Autodesk Inventor part; units mm, degrees
(part 2 of 2)
  line L146 (-17.2139, 92.4267) -> (-17.7029, 92.4267)
  line L147 (-17.7029, 92.4267) -> (-17.7029, 93.0096)
  line L148 (-20.1977, 93.0096) -> (-18.318, 93.0096)
  line L149 (-18.318, 93.0096) -> (-18.318, 92.5774)
  spline S117 degree 2 poles (-18.318, 92.5774) (-18.5205, 92.3872) (-18.8811, 92.034) (-19.054, 91.8438) knots 0 0 0 1 2 2 2
  spline S118 degree 2 poles (-19.054, 91.8438) (-19.4023, 91.4609) (-19.6567, 91.0015) (-19.6567, 90.757) knots 0 0 0 1 2 2 2
  spline S119 degree 2 poles (-19.6567, 90.757) (-19.6567, 90.6285) (-19.5777, 90.4359) (-19.5061, 90.3741) knots 0 0 0 1 2 2 2
  spline S120 degree 2 poles (-19.5061, 90.3741) (-19.4344, 90.3124) (-19.2467, 90.2506) (-19.1331, 90.2506) knots 0 0 0 1 2 2 2
  spline S121 degree 2 poles (-19.1331, 90.2506) (-19.0244, 90.2506) (-18.8021, 90.305) (-18.7008, 90.347) knots 0 0 0 1 2 2 2
  spline S122 degree 2 poles (-18.7008, 90.347) (-18.6144, 90.3815) (-18.4538, 90.4803) (-18.4044, 90.5149) knots 0 0 0 1 2 2 2
  line L150 (-18.4044, 90.5149) -> (-18.3822, 90.5149)
  line L151 (-18.3822, 90.5149) -> (-18.3822, 90.0802)
  spline S123 degree 2 poles (-18.3822, 90.0802) (-18.5082, 90.0184) (-18.9602, 89.8974) (-19.1627, 89.8974) knots 0 0 0 1 2 2 2
  spline S124 degree 2 poles (-19.1627, 89.8974) (-19.59, 89.8974) (-20.0717, 90.3494) (-20.0717, 90.7347) knots 0 0 0 1 2 2 2
  spline S125 degree 2 poles (-20.0717, 90.7347) (-20.0717, 90.9151) (-19.9877, 91.2164) (-19.9136, 91.3448) knots 0 0 0 1 2 2 2
  spline S126 degree 2 poles (-19.9136, 91.3448) (-19.8395, 91.4782) (-19.6246, 91.74) (-19.5061, 91.866) knots 0 0 0 1 2 2 2
  spline S127 degree 2 poles (-19.5061, 91.866) (-19.3134, 92.076) (-18.8416, 92.5255) (-18.7008, 92.6564) knots 0 0 0 1 2 2 2
  line L152 (-18.7008, 92.6564) -> (-20.1977, 92.6564)
  line L153 (-20.1977, 92.6564) -> (-20.1977, 93.0096)
  spline S128 degree 2 poles (-22.4528, 92.0414) (-22.4528, 92.2612) (-22.312, 92.6367) (-22.1836, 92.775) knots 0 0 0 1 2 2 2
  spline S129 degree 2 poles (-22.1836, 92.775) (-22.0551, 92.9133) (-21.6723, 93.0738) (-21.4351, 93.0738) knots 0 0 0 1 2 2 2
  spline S130 degree 2 poles (-21.4351, 93.0738) (-21.2178, 93.0738) (-20.7929, 92.9775) (-20.6373, 92.9009) knots 0 0 0 1 2 2 2
  line L154 (-20.6373, 92.9009) -> (-20.6373, 92.4687)
  line L155 (-20.6373, 92.4687) -> (-20.667, 92.4687)
  spline S131 degree 2 poles (-20.667, 92.4687) (-20.7139, 92.5033) (-20.8893, 92.5922) (-20.9955, 92.6317) knots 0 0 0 1 2 2 2
  spline S132 degree 2 poles (-20.9955, 92.6317) (-21.1165, 92.6737) (-21.3166, 92.7206) (-21.4426, 92.7206) knots 0 0 0 1 2 2 2
  spline S133 degree 2 poles (-21.4426, 92.7206) (-21.5661, 92.7206) (-21.7982, 92.6317) (-21.8822, 92.5354) knots 0 0 0 1 2 2 2
  spline S134 degree 2 poles (-21.8822, 92.5354) (-21.9588, 92.444) (-22.0378, 92.2019) (-22.0378, 92.0389) knots 0 0 0 1 2 2 2
  spline S135 degree 2 poles (-22.0378, 92.0389) (-22.0378, 91.8759) (-21.9489, 91.6684) (-21.8649, 91.5992) knots 0 0 0 1 2 2 2
  spline S136 degree 2 poles (-21.8649, 91.5992) (-21.7785, 91.5227) (-21.5216, 91.4585) (-21.366, 91.4585) knots 0 0 0 1 2 2 2
  spline S137 degree 2 poles (-21.366, 91.4585) (-21.198, 91.4585) (-20.8646, 91.5103) (-20.7633, 91.5326) knots 0 0 0 1 2 2 2
  line L156 (-20.7633, 91.5326) -> (-20.7633, 89.9616)
  line L157 (-20.7633, 89.9616) -> (-22.4355, 89.9616)
  line L158 (-22.4355, 89.9616) -> (-22.4355, 90.3198)
  line L159 (-22.4355, 90.3198) -> (-21.156, 90.3198)
  line L160 (-21.156, 90.3198) -> (-21.156, 91.1324)
  spline S138 degree 2 poles (-21.156, 91.1324) (-21.2301, 91.1225) (-21.3734, 91.1151) (-21.4327, 91.1151) knots 0 0 0 1 2 2 2
  spline S139 degree 2 poles (-21.4327, 91.1151) (-21.6673, 91.1151) (-21.9909, 91.1917) (-22.1391, 91.3053) knots 0 0 0 1 2 2 2
  spline S140 degree 2 poles (-22.1391, 91.3053) (-22.2898, 91.4189) (-22.4528, 91.7647) (-22.4528, 92.0414) knots 0 0 0 1 2 2 2
  point P0 (-47.5, 53.2457)
  constraints: 2 other
extrude "Extrusion47" cut sketch "Sketch58" against normal blind 1.5
sketch "Sketch59" plane through (69.5, 80.5, 0) normal (0, 0, -1) x (-1, 0, 0)
  line L0 (124.232, -148.2248) -> (124.232, -65.5994) projected
  line L1 (124.232, -131.7625) -> (22.225, -131.7625)
  line L2 (22.225, -144.4625) -> (124.232, -144.4625)
  line L3 (124.232, -144.4625) -> (124.232, -131.7625)
  line L4 (22.225, -144.4625) -> (19.05, -144.4625)
  line L5 (19.05, -144.4625) -> (19.05, -131.7625)
  line L6 (19.05, -131.7625) -> (22.225, -131.7625)
  point P0 (69.5, -80.5)
  point P1 (22.225, -131.7625)
  constraints: 12 end point, 2 horizontal, 2 parallel, 1 perpendicular, 1 point on line
extrude "Extrusion48" add sketch "Sketch59" against normal blind 1
sketch "Sketch61" plane through (-54.732, -66.7303, 5) normal (-1, 0, 0) x (0, 0, 1)
  point P0 (-5, 66.7303)
sketch "Sketch63" plane through (-54.732, -66.7303, 5) normal (-1, 0, 0) x (0, 0, 1)
  line L0 (0, 0) -> (32.8849, -46.9646) projected
  line L1 (32.8849, -46.9646) -> (72.2795, -19.3802)
  line L2 (72.2795, -19.3802) -> (86.4989, -39.6875)
  line L3 (86.4989, -39.6875) -> (32.8849, -46.9646)
  point P0 (-5, 66.7303)
  constraints: 6 end point, 2 perpendicular
extrude "Extrusion50" cut sketch "Sketch63" against normal blind 155.1
sketch "Sketch64" plane through (-54.732, -87.3593, 75.4961) normal (0, -0.819152, 0.5735764) x (1, 0, 0)
  line L0 (6, 0) -> (6, -45.9148) projected
  line L1 (0, -45.9148) -> (0, 21.0852) projected
  line L2 (0, 0) -> (0, -5)
  line L3 (0, -5) -> (3.5, -5)
  line L4 (3.5, -5) -> (0.6132, 0)
  line L5 (0, 0) -> (0, 0.5341)
  line L6 (0, 0.5341) -> (0.3049, 0.5341)
  line L7 (0.3049, 0.5341) -> (0.6312, -0.0311)
  line L8 (98.464, 0) -> (104.464, 0) projected
  line L9 (104.464, 0) -> (104.464, -5)
  line L10 (104.464, 21.0852) -> (104.464, -45.9148) projected
  line L11 (104.464, -5) -> (100.964, -5)
  line L12 (100.964, -5) -> (103.8508, 0)
  line L13 (103.8508, 0) -> (104.1591, 0.5341)
  line L14 (104.1591, 0.5341) -> (104.464, 0.5341)
  line L15 (104.464, 0.5341) -> (104.464, -0.2668)
  point P0 (0.6132, 0)
  dimension "d248" = 5
  dimension "d249" = 3.5
  dimension "d250" = 60
  dimension "d251" = 5
  dimension "d252" = 3.5
  dimension "d253" = 60
  constraints: 24 end point, 7 point on line, 2 horizontal, 2 perpendicular
  measures "d248" distance of L2.start L2.end
  measures "d249" distance of L2.end L3.end
  measures "d250" angle of L4 L3
  measures "d251" distance of L8.end L9.end
  measures "d252" distance of L9.end L11.end
  measures "d253" angle of L12 L11
extrude "Extrusion51" cut sketch "Sketch64" against normal blind 100.764
sketch "Sketch65" plane through (47.5, -63.2207, 2.5425) normal (0, -0.5735764, -0.819152) x (-1, 0, 0)
  circle A0 centre (74.6125, -57.15) radius 2 projected
  circle A1 centre (74.6125, -57.15) radius 5
  circle A2 centre (84.6125, -33.45) radius 2 projected
  circle A3 centre (84.6125, -33.45) radius 5
  circle A4 centre (64.6125, -33.45) radius 2 projected
  circle A5 centre (64.6125, -33.45) radius 5
  point P0 (47.5, 53.2457)
  dimension "d254" = 10
  dimension "d255" = 10
  dimension "d256" = 10
  constraints: 3 centre point, 3 coincident
  measures "d254" diameter of A1
  measures "d255" diameter of A3
  measures "d256" diameter of A5
extrude "Extrusion52" cut sketch "Sketch65" against normal blind 3 contours A1 | A2 | A3 | A4 | A5
sketch "Sketch66" plane through (-48.732, -55.8368, 7.1384) normal (0, 0.819152, -0.5735764) x (1, 0, 0)
  line L0 (42.232, 0) -> (42.232, -16) projected
  line L1 (0, 0) -> (42.232, 0) projected
  line L2 (0, -16) -> (0, 0)
  line L3 (0, 0) -> (42.232, 0)
  line L4 (42.232, 0) -> (42.232, -16)
  arc A0 (34.925, -16) -> (9.0575, -16) centre (21.9913, -30.5193) ccw projected
  arc A1 (34.925, -16) -> (9.0575, -16) centre (21.9913, -30.5193) ccw
  line L5 (42.232, -16) -> (34.925, -16)
  line L6 (9.0575, -16) -> (0, -16)
  point P0 (48.732, -26.1792)
  constraints: 10 end point, 4 point on circle, 3 parallel, 2 horizontal, 2 perpendicular, 1 centre point
extrude "Extrusion53" add sketch "Sketch66" along normal blind 2
sketch "Sketch67" plane through (47.5, -58.6321, 9.0958) normal (0, 0.5735764, 0.819152) x (1, 0, 0)
  line L0 (-96.232, 5.4125) -> (-96.232, 15.858) projected
  line L1 (-3.768, -61.6176) -> (-3.768, 39.1469) projected
  line L2 (-3.768, 5.4125) -> (-3.768, 15.875)
  line L3 (-3.768, 15.875) -> (-96.232, 15.875)
  line L4 (-96.232, 15.875) -> (-96.232, 5.4125)
  line L5 (-3.768, 10.6437) -> (-96.232, 10.6437)
  point P0 (-47.5, 53.2457)
  point P1 (-96.232, 15.858)
  point P2 (-3.768, 10.6437)
  constraints: 8 end point, 2 midpoint, 1 parallel, 1 point on line
extrude "Extrusion54" add sketch "Sketch67" along normal blind 50
sketch "Sketch70" plane through (-48.732, -45.6281, -0.0098) normal (0, 0.819152, -0.5735764) x (1, 0, 0)
  line L0 (92.464, -37.9148) -> (92.464, -50) projected
  line L1 (0, -0.0119) -> (0, -60) projected
  line L2 (92.464, -50) -> (0, -50)
  line L3 (0, -50) -> (0, -0.0119)
  line L4 (0, -0.0119) -> (92.464, -0.0119)
  line L5 (92.464, -0.0119) -> (92.464, -50)
  point P0 (48.732, -26.1792)
  point P1 (0, -50)
  constraints: 8 end point, 2 parallel, 1 horizontal, 1 perpendicular
extrude "Extrusion57" add sketch "Sketch70" along normal blind 10
sketch "Sketch72" plane through (47.5, -29.9533, 50.0534) normal (0, 0.5735764, 0.819152) x (1, 0, 0)
  line L0 (-96.232, 39.1469) -> (-96.232, 25.875) projected
  line L1 (-3.768, 10.6438) -> (-3.768, 25.875) projected
  line L2 (-96.232, 25.875) -> (-3.768, 25.875)
  line L3 (-3.768, 25.875) -> (-3.768, 10.6438)
  line L4 (-3.768, 10.6438) -> (-96.232, 10.6438)
  line L5 (-96.232, 10.6438) -> (-96.232, 25.875)
  point P0 (-47.5, 53.2457)
  point P1 (-3.768, 25.875)
  constraints: 8 end point, 2 parallel, 1 horizontal, 1 perpendicular
extrude "Extrusion59" add sketch "Sketch72" along normal blind 10
sketch "Sketch75" plane through (-48.732, -45.6212, 0) normal (-1, 0, 0) x (0, 0, 1)
  line L0 (0, 126.1212) -> (0, -24.1778) projected
  line L1 (0, 17.4625) -> (-11.1125, 17.4625)
  line L2 (-11.1125, 17.4625) -> (-11.1125, -14.2875)
  line L3 (-11.1125, -14.2875) -> (0, -14.2875)
  line L4 (0, -14.2875) -> (0, 17.4625)
  point P0 (0, 45.6212)
  point P1 (0, -14.2875)
  constraints: 8 end point, 2 parallel, 1 horizontal, 1 perpendicular, 1 point on line
extrude "Extrusion60" cut sketch "Sketch75" against normal through all
sketch "Sketch76" plane through (-48.732, -49.9133, 2.9908) normal (0, -0.819152, 0.5735764) x (1, 0, 0)
  circle A0 centre (66.464, 37.5) radius 17
  line L0 (92.464, 37.9148) -> (92.464, 0) projected
  line L1 (92.464, 0) -> (0, 0) projected
  point P0 (48.732, 26.1792)
  dimension "d279" = 34
  dimension "d280" = 26
  dimension "d281" = 37.5
  constraints: 1 centre point
  measures "d279" diameter of A0
  measures "d280" distance from line of L0 A0.centre
  measures "d281" distance from line of A0.centre L1
extrude "Extrusion61" cut sketch "Sketch76" against normal through all
sketch "Sketch77" plane through (-48.732, -37.4366, -5.7455) normal (0, 0.819152, -0.5735764) x (1, 0, 0)
  circle A0 centre (21.62, -30.5) radius 20
  line L0 (92.464, -7.014) -> (0, -7.014) projected
  line L1 (0, -60) -> (92.464, -60) projected
  line L2 (0, -7.014) -> (0, -60) projected
  point P0 (48.732, -26.1792)
  dimension "d284" = 40
  dimension "d287" = 29.5
  dimension "d288" = 21.62
  constraints: 1 centre point
  measures "d284" diameter of A0
  measures "d287" distance from line of L1 A0.centre
  measures "d288" distance from line of L2 A0.centre
extrude "Extrusion62" cut sketch "Sketch77" against normal blind 16
body "Solid1"
